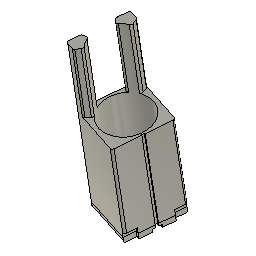
Battery Holder v27 (Autodesk Fusion 360 design; units mm, degrees)
Autodesk Fusion 360 part; units mm, degrees
sketch "Sketch1" plane through (0, 0, 0) normal (0, 0, 1) x (1, 0, 0)
  line L0 (18, 19.15) -> (-18, 19.15)
  line L1 (-18, 19.15) -> (-18, -19.15)
  line L2 (-18, -19.15) -> (18, -19.15)
  line L3 (18, -19.15) -> (18, 19.15)
  line L4 (18, 19.15) -> (-18, -19.15) construction
  line L5 (-18, 19.15) -> (18, -19.15) construction
  circle A0 centre (0, 0) radius 16.5
  circle A1 centre (0, 0) radius 5
  circle A2 centre (0, 0) radius 2.5
  dimension "d1" = 36
  dimension "d2" = 38.3
  dimension "d3" = 33
  dimension "d14" = 10
  dimension "d98" = 5
  constraint horizontal L0
  constraint perpendicular L0 L1
  constraint parallel L0 L2
  constraint parallel L1 L3
  constraint coincident L4 A0.centre
  constraint coincident L5 A0.centre
  constraint coincident A0.centre A1.centre
  measures "d1" distance of L1.end L2.end
  measures "d2" distance of L0.end L1.end
  measures "d3" diameter of A0
  measures "d14" diameter of A1
  measures "d98" diameter of A2
extrude "Extrude1" add sketch "Sketch1" along normal blind 65 contours L0 L1 L2 L3 makes body 1
extrude "Extrude2" add sketch "Sketch1" against normal blind 4 separate body contours L0 L1 L2 L3 | A0 | A1 | A2 makes body 2
extrude "Extrude3" cut sketch "Sketch1" against normal up to surface (4 mm away) contours A1 | A2 bodies 2
sketch "Sketch2" plane through (0, 0, -4) normal (0, 0, -1) x (1, 0, 0)
  circle A0 centre (0, 0) radius 5
  line L0 (18, -19.15) -> (18, 19.15)
  line L1 (18, 19.15) -> (-18, 19.15)
  line L2 (-18, 19.15) -> (-18, -19.15)
  line L3 (-18, -19.15) -> (18, -19.15)
  line L4 (18, 19.15) -> (16, 19.15)
  line L5 (16, 19.15) -> (16, 11.15)
  line L6 (16, 11.15) -> (18, 11.15)
  line L7 (18, 11.15) -> (18, 19.15)
  line L8 (18, -19.15) -> (16, -19.15)
  line L9 (16, -19.15) -> (16, -11.15)
  line L10 (16, -11.15) -> (18, -11.15)
  line L11 (18, -11.15) -> (18, -19.15)
  line L12 (18, -3) -> (0, -3)
  line L13 (0, -3) -> (0, 3)
  line L14 (0, 3) -> (18, 3)
  line L15 (18, 3) -> (18, -3)
  dimension "d19" = 2
  dimension "d20" = 8
  dimension "d28" = 36
  dimension "d29" = 38.3
  dimension "d30" = 2
  dimension "d31" = 8
  dimension "d38" = 6
  constraint horizontal L4
  constraint vertical L5
  constraint horizontal L6
  constraint vertical L7
  constraint coincident L0.end L1.start
  constraint horizontal L8
  constraint vertical L9
  constraint horizontal L10
  constraint vertical L11
  constraint coincident L0.start L3.end
  constraint horizontal L12
  constraint vertical L13
  constraint horizontal L14
  constraint midpoint A0.centre L13
  constraint collinear L0 L15
  measures "d19" distance of L5.end L6.end
  measures "d20" distance of L4.end L5.end
  measures "d28" distance of L0.start L2.end
  measures "d29" distance of L1.end L2.end
  measures "d30" distance of L9.end L10.end
  measures "d31" distance of L0.start L10.end
  measures "d38" distance of L12 L14
extrude "Extrude4" cut sketch "Sketch2" against normal blind 8 contours L0 L1 L4 L5 L6 L7 bodies 1 2
extrude "Extrude5" cut sketch "Sketch2" against normal blind 8 contours L0 L3 L8 L9 L10 L11 bodies 1 2
extrude "Extrude7" cut sketch "Sketch2" against normal blind 2 contours A0 L0 L12 L14 L15 bodies 2
fillet "Fillet1" radius 2 1 edges at (5, 0, -2) on bodies 2
sketch "Sketch3" plane through (18, 0, 0) normal (1, 0, 0) x (0, 1, 0)
  line L0 (11.15, 0) -> (11.15, 4)
  line L1 (11.15, 4) -> (19.15, 4)
  line L2 (19.15, 4) -> (19.15, 65)
  line L3 (19.15, 65) -> (-19.15, 65)
  line L4 (-19.15, 65) -> (-19.15, 4)
  line L5 (-19.15, 4) -> (-11.15, 4)
  line L6 (-11.15, 4) -> (-11.15, 0)
  line L7 (-11.15, 0) -> (11.15, 0)
  line L8 (1, -4) -> (1, 65)
  line L9 (1, 65) -> (-1, 65)
  line L10 (-1, 65) -> (-1, -4.0808)
  line L11 (-3, -2) -> (3, -2)
  line L12 (1, -4) -> (-1, -4.0808)
  dimension "d43" = 2
  dimension "d49" = 69
  constraint vertical L8
  constraint horizontal L9
  constraint vertical L10
  constraint coincident L3 L8.end
  constraint midpoint L3 L9
  measures "d43" distance of L8.end L9.end
  measures "d49" distance of L8.start L8.end
extrude "Extrude9" cut sketch "Sketch3" against normal blind 0.5 contours L7 L8 L10 L11 | L3 L7 L8 L9 L10 bodies 1 2
fillet "Fillet2" radius 3 1 edges at (17.5, 0, -2) on bodies 2
sketch "Sketch4" plane through (0, 0, 65) normal (0, 0, 1) x (-1, 0, 0)
  line L0 (-18, 1) -> (-17.5, 1)
  line L1 (-17.5, 1) -> (-17.5, -1)
  line L2 (-17.5, -1) -> (-18, -1)
  line L3 (-18, -1) -> (-18, -19.15)
  line L4 (-18, -19.15) -> (18, -19.15)
  line L5 (18, -19.15) -> (18, 19.15)
  line L6 (18, 19.15) -> (-18, 19.15)
  line L7 (-18, 19.15) -> (-18, 1)
  circle A0 centre (0, 0) radius 16.5
  circle A1 centre (0, 0) radius 16.5
  line L8 (0, 26.0938) -> (0, -34.6828) construction
  line L9 (23.92, 0) -> (-29.2595, 0) construction
  line L10 (0, 0) -> (1.2207, 0)
  line L11 (0, 0) -> (11.0877, 19.2044)
  line L12 (11.0563, 19.15) -> (18, 19.15)
  line L13 (0, 0) -> (18, 10.3923)
  line L14 (18, 19.15) -> (18, 10.3923)
  line L15 (18, -19.15) -> (-18, -19.15)
  line L16 (-18, -19.15) -> (-18, 19.15)
  line L17 (-18, 19.15) -> (18, 19.15)
  line L18 (18, 19.15) -> (18, -19.15)
  line L19 (0, 0) -> (18, -10.3923)
  line L20 (0, 0) -> (11.0563, -19.15)
  dimension "d86" = 33
  dimension "d109" = 36
  dimension "d110" = 38.3
  dimension "d111" = 30
  dimension "d116" = 30
  dimension "d117" = 30
  dimension "d118" = 30
  constraint coincident A0.centre A1.centre
  constraint vertical L8
  constraint perpendicular L1 L9
  constraint coincident L9 L10.end
  constraint coincident L11 L12.start
  constraint coincident L6 L12.start
  constraint coincident L5.end L6.start
  constraint coincident L13 L14.end
  constraint coincident L5 L13.end
  constraint horizontal L15
  constraint vertical L16
  constraint horizontal L17
  constraint vertical L18
  constraint coincident L6.end L7.start
  constraint coincident L4.end L5.start
  constraint coincident L4 L20.end
  constraint coincident L18 L19.end
  measures "d86" diameter of A1
  measures "d109" distance of L5.end L6.end
  measures "d110" distance of L4.end L5.end
  measures "d111" angle of L8 L11
  measures "d116" angle of L9 L13
  measures "d117" angle of L8 L20
  measures "d118" angle of L9 L19
sketch "Sketch5" plane through (0, 19.15, 0) normal (0, 1, 0) x (-1, 0, 0)
  line L0 (-16, 4) -> (-16, 0)
  line L1 (-16, 0) -> (18, 0)
  line L2 (18, 0) -> (18, 65)
  line L3 (18, 65) -> (-18, 65)
  line L4 (-18, 65) -> (-18, 4)
  line L5 (-18, 4) -> (-16, 4)
  line L6 (-0.75, 16) -> (0.75, 16)
  line L7 (0.75, 16) -> (0.75, 6)
  line L8 (0.75, 6) -> (-0.75, 6)
  line L9 (-0.75, 6) -> (-0.75, 16)
  line L10 (-5, 11.75) -> (5, 11.75)
  line L11 (5, 11.75) -> (5, 10.25)
  line L12 (5, 10.25) -> (-5, 10.25)
  line L13 (-5, 10.25) -> (-5, 11.75)
  line L14 (-23.8589, 11) -> (22.3589, 11) construction
  line L15 (0.75, 59) -> (-0.75, 59)
  line L16 (-0.75, 59) -> (-0.75, 49)
  line L17 (-0.75, 49) -> (0.75, 49)
  line L18 (0.75, 49) -> (0.75, 59)
  dimension "d60" = 1.5
  dimension "d61" = 10
  dimension "d62" = 6
  dimension "d63" = 17.25
  dimension "d64" = 1.5
  dimension "d65" = 10
  dimension "d66" = 13
  dimension "d67" = 11
  dimension "d68" = 0.75
  dimension "d71" = 10
  dimension "d72" = 1.5
  dimension "d73" = 6
  constraint horizontal L6
  constraint vertical L7
  constraint horizontal L8
  constraint vertical L9
  constraint horizontal L10
  constraint vertical L11
  constraint horizontal L12
  constraint vertical L13
  constraint perpendicular L2 L14
  constraint midpoint L9 L14
  constraint horizontal L15
  constraint vertical L16
  constraint horizontal L17
  constraint vertical L18
  constraint collinear L9 L16
  measures "d60" distance of L6.start L6.end
  measures "d61" distance of L6.start L8.end
  measures "d62" distance of L1 L8
  measures "d63" distance of L4 L9
  measures "d64" distance of L10.end L11.end
  measures "d65" distance of L10.start L10.end
  measures "d66" distance of L4 L13
  measures "d67" distance of L1 L14
  measures "d68" distance of L10 L14
  measures "d71" distance of L15.start L17.end
  measures "d72" distance of L15.start L15.end
  measures "d73" distance of L3 L15
extrude "Extrude11" cut sketch "Sketch5" against normal blind 0.2 contours L6 L7 L9 L10 | L7 L9 L10 L12 | L9 L10 L12 L13 | L7 L10 L11 L12 | L7 L8 L9 L12 | L15 L16 L17 L18 bodies 1
fillet "Fillet3" radius 0.2 2 edges at (17.5, 1, 32.5) (17.5, -1, 32.5) on bodies 1
copy_body "Body->Comp1" bodies 1 removing the originals makes body 3 in component "Holder"
copy_body "Body->Comp2" bodies 2 removing the originals makes body 4 in component "Base"
fillet "Fillet3'" radius 1.5 2 edges at (-18, -19.15, -2) (-18, 19.15, -2) on bodies 4 in component "Base"
fillet "Fillet2'" radius 1.5 4 edges at (18, 19.15, 34.5) (18, -19.15, 34.5) (-18, -19.15, 32.5) (-18, 19.15, 32.5) on bodies 3 in component "Holder"
extrude "Extrude14" add sketch "Sketch1" along normal blind 60 separate body contours A0 | A1 | A2 makes body 5
extrude "Extrude15" add sketch "Sketch1" against normal blind 2 contours A2 bodies 5
copy_body "Body->Comp4" bodies 5 removing the originals makes body 6 in component "Battery (1)"
extrude "Extrude2'" add sketch "Sketch4" along normal blind 49.7 contours L5 L6 A0 A1 L11 L12 L13 L14 L17 L18 | L4 L5 A0 A1 L15 L18 L19 L20 bodies 3 in component "Holder"
fillet "Fillet5" radius 1.5 4 edges at (-8.25, -14.2894, 89.85) (-14.2894, -8.25, 89.85) (-14.2894, 8.25, 89.85) (-8.25, 14.2894, 89.85) on bodies 3 in component "Holder"
fillet "Fillet5" radius 1.5 4 edges at (-18, 19.15, 89.85) (-18, 10.3923, 89.85) (-18, -10.3923, 89.85) (-18, -19.15, 89.85) on bodies 3 in component "Holder"
fillet "Fillet5" radius 1.5 2 edges at (-11.0563, 19.15, 89.85) (-11.0563, -19.15, 89.85) on bodies 3 in component "Holder"
fillet "Fillet4" radius 1.5 5 edges at (-0.25, -19.15, -4) (-17.5607, -18.7107, -4) (-18, 0, -4) (-17.5607, 18.7107, -4) (-0.25, 19.15, -4) on bodies 4 in component "Base"
extrude "Extrude12" [suppressed]
extrude "Extrude13" [suppressed]
copy_body "Body->Comp3" [suppressed] in component "Battery"
component "Holder" placed x (1, 0, 0) y (0, 1, 0) z (0, 0, 1) at (0, 0, 0)
component "Base" placed x (1, 0, 0) y (0, 1, 0) z (0, 0, 1) at (0, 0, 0)
component "Battery (1)" placed x (1, 0, 0) y (0, 1, 0) z (0, 0, 1) at (0, 0, 0)
equation "d1 = BaseWidth"
equation "d2 = BaseHeight"
equation "d3 = BatteryHoleDia"
equation "d4 = BatteryHoleLength"
equation "BaseWidth = 36 mm"
equation "BatteryHoleDia = 33 mm"
equation "LengthOverAll = 118.7 mm"
equation "BatteryHoleLength = 65 mm"
equation "BaseThickness = 4 mm"
equation "d11 = -BaseThickness"
equation "TerminalHoleDia = 10 mm"
equation "d14 = TerminalHoleDia"
equation "CutoutHeight = 8 mm"
equation "CutoutWidth = 2 mm"
equation "d19 = CutoutWidth"
equation "d20 = CutoutHeight"
equation "BaseHeight = 38.3 mm"
equation "d30 = CutoutWidth"
equation "d31 = CutoutHeight"
equation "GrooveWidth = 6 mm"
equation "GrooveDepth = 2 mm"
equation "d38 = GrooveWidth"
equation "d39 = -GrooveDepth"
equation "d49 = BatteryHoleLength + BaseThickness"
equation "d63 = ( BaseWidth - 1.5 mm ) / 2"
equation "d64 = d60"
equation "d65 = d61"
equation "d66 = ( BaseWidth - d65 ) / 2"
equation "d68 = d64 / 2"
equation "d71 = d61"
equation "d72 = d60"
equation "d73 = d62"
equation "d119 = LengthOverAll - BatteryHoleLength - BaseThickness"
